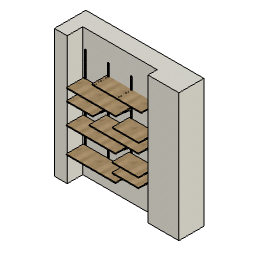
shelving_system (Autodesk Fusion 360 design; units mm, degrees)
Autodesk Fusion 360 part; units mm, degrees
note: some values were not read from the file. Chosen so that the rebuilt part matches the saved one: which face or edge a step refers to; the sign of a taper; where a step ends.
sketch "Sketch1" plane through (0, 0, 0) normal (0, 1, 0) x (1, 0, 0)
  line L0 (0, 0) -> (26, 0)
  line L1 (26, 0) -> (26, -1995)
  line L2 (26, -1995) -> (0, -1995)
  line L3 (0, -1995) -> (0, 0)
  dimension "d1" = 26
  dimension "d2" = 1995
  constraint horizontal L0
  constraint vertical L1
  constraint horizontal L2
  constraint vertical L3
  constraint coincident L0.start L3.end
  measures "d1" distance of L0.start L0.end
  measures "d2" distance of L0.start L2.end
extrude "Extrude1" add sketch "Sketch1" along normal blind 12 makes body 1
sketch "Sketch2" plane through (0, 0, 0) normal (0, -1, 0) x (1, 0, 0)
  line L0 (26, 1995) -> (0, 1995)
  line L1 (0, 1995) -> (0, 0)
  line L2 (0, 0) -> (26, 0)
  line L3 (26, 0) -> (26, 1995)
  line L4 (6.3705, 1487.1399) -> (6.3705, 1462.1399)
  arc A0 (6.3705, 1462.1399) -> (9.3705, 1462.1399) centre (7.8705, 1462.1399) ccw
  line L5 (9.3705, 1462.1399) -> (9.3705, 1487.1399)
  arc A1 (9.3705, 1487.1399) -> (6.3705, 1487.1399) centre (7.8705, 1487.1399) ccw
  line L6 (7.8705, 1487.1399) -> (7.8705, 1462.1399) construction
  dimension "d5" = 3
  constraint tangent L4 A0
  constraint tangent A0 L5
  constraint parallel L4 L5
  constraint tangent L5 A1
  constraint tangent L4 A1
  constraint vertical L6
  measures "d5" diameter of A0
extrude "Extrude2" cut sketch "Sketch2" along normal up to far side of body 1 contours L4 A0 L5 A1 bodies 1
ref_plane "WorkPlane1" through (13, 6, 997.5) normal (-1, 0, 0) x (0, 0, 1)
mirror "Mirror1" about plane through (13, 6, 997.5) normal (-1, 0, 0) of "Extrude2"
pattern_linear "R-Pattern1" count 30 spacing 50 along (0, 0, -1) of 8 faces at (6.3705, 4, 1478.8066) (9.3705, 4, 1470.4732) (6.878, 8, 1461.0152) (6.878, 4, 1488.2646) (19.6295, 4, 1478.8066) (16.6295, 4, 1470.4732) (17.137, 8, 1488.2646) (19.122, 8, 1461.0152) on bodies 1
pattern_linear "R-Pattern3" count 11 spacing 50 along (0, 0, 1) of 8 faces at (6.878, 4, 1488.2646) (6.3705, 4, 1478.8066) (9.3705, 4, 1470.4732) (17.137, 8, 1488.2646) (6.878, 8, 1461.0152) (19.6295, 4, 1478.8066) (16.6295, 4, 1470.4732) (19.122, 8, 1461.0152) on bodies 1
pattern_linear "R-Pattern2" count 4 spacing 500 along (1, 0, 0) of bodies 1 makes body 2 at (511.5402, 0, 3.6136) makes body 3 at (1011.5402, 0, 3.6136) makes body 4 at (1511.5402, 0, 3.6136)
sketch "Sketch3" plane through (0, 0, 0) normal (0, -1, 0) x (1, 0, 0)
  line L0 (16.6295, 12.1399) -> (16.6295, 37.1399)
  arc A0 (19.6295, 37.1399) -> (16.6295, 37.1399) centre (18.1295, 37.1399) ccw
  line L1 (19.6295, 37.1399) -> (19.6295, 12.1399)
  arc A1 (16.6295, 12.1399) -> (19.6295, 12.1399) centre (18.1295, 12.1399) ccw
  line L2 (16.6295, 62.1399) -> (16.6295, 87.1399)
  arc A2 (19.6295, 87.1399) -> (16.6295, 87.1399) centre (18.1295, 87.1399) ccw
  line L3 (19.6295, 87.1399) -> (19.6295, 62.1399)
  arc A3 (16.6295, 62.1399) -> (19.6295, 62.1399) centre (18.1295, 62.1399) ccw
  line L4 (16.6295, 112.1399) -> (16.6295, 137.1399)
  arc A4 (19.6295, 137.1399) -> (16.6295, 137.1399) centre (18.1295, 137.1399) ccw
  line L5 (19.6295, 137.1399) -> (19.6295, 112.1399)
  arc A5 (16.6295, 112.1399) -> (19.6295, 112.1399) centre (18.1295, 112.1399) ccw
  line L6 (16.6295, 162.1399) -> (16.6295, 187.1399)
  arc A6 (19.6295, 187.1399) -> (16.6295, 187.1399) centre (18.1295, 187.1399) ccw
  line L7 (19.6295, 187.1399) -> (19.6295, 162.1399)
  arc A7 (16.6295, 162.1399) -> (19.6295, 162.1399) centre (18.1295, 162.1399) ccw
  line L8 (16.6295, 212.1399) -> (16.6295, 237.1399)
  arc A8 (19.6295, 237.1399) -> (16.6295, 237.1399) centre (18.1295, 237.1399) ccw
  line L9 (19.6295, 237.1399) -> (19.6295, 212.1399)
  arc A9 (16.6295, 212.1399) -> (19.6295, 212.1399) centre (18.1295, 212.1399) ccw
  line L10 (16.6295, 262.1399) -> (16.6295, 287.1399)
  arc A10 (19.6295, 287.1399) -> (16.6295, 287.1399) centre (18.1295, 287.1399) ccw
  line L11 (19.6295, 287.1399) -> (19.6295, 262.1399)
  arc A11 (16.6295, 262.1399) -> (19.6295, 262.1399) centre (18.1295, 262.1399) ccw
  line L12 (16.6295, 312.1399) -> (16.6295, 337.1399)
  arc A12 (19.6295, 337.1399) -> (16.6295, 337.1399) centre (18.1295, 337.1399) ccw
  line L13 (19.6295, 337.1399) -> (19.6295, 312.1399)
  arc A13 (16.6295, 312.1399) -> (19.6295, 312.1399) centre (18.1295, 312.1399) ccw
  line L14 (16.6295, 362.1399) -> (16.6295, 387.1399)
  arc A14 (19.6295, 387.1399) -> (16.6295, 387.1399) centre (18.1295, 387.1399) ccw
  line L15 (19.6295, 387.1399) -> (19.6295, 362.1399)
  arc A15 (16.6295, 362.1399) -> (19.6295, 362.1399) centre (18.1295, 362.1399) ccw
  line L16 (16.6295, 412.1399) -> (16.6295, 437.1399)
  arc A16 (19.6295, 437.1399) -> (16.6295, 437.1399) centre (18.1295, 437.1399) ccw
  line L17 (19.6295, 437.1399) -> (19.6295, 412.1399)
  arc A17 (16.6295, 412.1399) -> (19.6295, 412.1399) centre (18.1295, 412.1399) ccw
  line L18 (16.6295, 462.1399) -> (16.6295, 487.1399)
  arc A18 (19.6295, 487.1399) -> (16.6295, 487.1399) centre (18.1295, 487.1399) ccw
  line L19 (19.6295, 487.1399) -> (19.6295, 462.1399)
  arc A19 (16.6295, 462.1399) -> (19.6295, 462.1399) centre (18.1295, 462.1399) ccw
  line L20 (16.6295, 512.1399) -> (16.6295, 537.1399)
  arc A20 (19.6295, 537.1399) -> (16.6295, 537.1399) centre (18.1295, 537.1399) ccw
  line L21 (19.6295, 537.1399) -> (19.6295, 512.1399)
  arc A21 (16.6295, 512.1399) -> (19.6295, 512.1399) centre (18.1295, 512.1399) ccw
  line L22 (16.6295, 562.1399) -> (16.6295, 587.1399)
  arc A22 (19.6295, 587.1399) -> (16.6295, 587.1399) centre (18.1295, 587.1399) ccw
  line L23 (19.6295, 587.1399) -> (19.6295, 562.1399)
  arc A23 (16.6295, 562.1399) -> (19.6295, 562.1399) centre (18.1295, 562.1399) ccw
  line L24 (16.6295, 612.1399) -> (16.6295, 637.1399)
  arc A24 (19.6295, 637.1399) -> (16.6295, 637.1399) centre (18.1295, 637.1399) ccw
  line L25 (19.6295, 637.1399) -> (19.6295, 612.1399)
  arc A25 (16.6295, 612.1399) -> (19.6295, 612.1399) centre (18.1295, 612.1399) ccw
  line L26 (16.6295, 662.1399) -> (16.6295, 687.1399)
  arc A26 (19.6295, 687.1399) -> (16.6295, 687.1399) centre (18.1295, 687.1399) ccw
  line L27 (19.6295, 687.1399) -> (19.6295, 662.1399)
  arc A27 (16.6295, 662.1399) -> (19.6295, 662.1399) centre (18.1295, 662.1399) ccw
  line L28 (16.6295, 712.1399) -> (16.6295, 737.1399)
  arc A28 (19.6295, 737.1399) -> (16.6295, 737.1399) centre (18.1295, 737.1399) ccw
  line L29 (19.6295, 737.1399) -> (19.6295, 712.1399)
  arc A29 (16.6295, 712.1399) -> (19.6295, 712.1399) centre (18.1295, 712.1399) ccw
  line L30 (16.6295, 762.1399) -> (16.6295, 787.1399)
  arc A30 (19.6295, 787.1399) -> (16.6295, 787.1399) centre (18.1295, 787.1399) ccw
  line L31 (19.6295, 787.1399) -> (19.6295, 762.1399)
  arc A31 (16.6295, 762.1399) -> (19.6295, 762.1399) centre (18.1295, 762.1399) ccw
  line L32 (16.6295, 812.1399) -> (16.6295, 837.1399)
  arc A32 (19.6295, 837.1399) -> (16.6295, 837.1399) centre (18.1295, 837.1399) ccw
  line L33 (19.6295, 837.1399) -> (19.6295, 812.1399)
  arc A33 (16.6295, 812.1399) -> (19.6295, 812.1399) centre (18.1295, 812.1399) ccw
  line L34 (16.6295, 862.1399) -> (16.6295, 887.1399)
  arc A34 (19.6295, 887.1399) -> (16.6295, 887.1399) centre (18.1295, 887.1399) ccw
  line L35 (19.6295, 887.1399) -> (19.6295, 862.1399)
  arc A35 (16.6295, 862.1399) -> (19.6295, 862.1399) centre (18.1295, 862.1399) ccw
  line L36 (16.6295, 912.1399) -> (16.6295, 937.1399)
  arc A36 (19.6295, 937.1399) -> (16.6295, 937.1399) centre (18.1295, 937.1399) ccw
  line L37 (19.6295, 937.1399) -> (19.6295, 912.1399)
  arc A37 (16.6295, 912.1399) -> (19.6295, 912.1399) centre (18.1295, 912.1399) ccw
  line L38 (16.6295, 962.1399) -> (16.6295, 987.1399)
  arc A38 (19.6295, 987.1399) -> (16.6295, 987.1399) centre (18.1295, 987.1399) ccw
  line L39 (19.6295, 987.1399) -> (19.6295, 962.1399)
  arc A39 (16.6295, 962.1399) -> (19.6295, 962.1399) centre (18.1295, 962.1399) ccw
  line L40 (16.6295, 1012.1399) -> (16.6295, 1037.1399)
  arc A40 (19.6295, 1037.1399) -> (16.6295, 1037.1399) centre (18.1295, 1037.1399) ccw
  line L41 (19.6295, 1037.1399) -> (19.6295, 1012.1399)
  arc A41 (16.6295, 1012.1399) -> (19.6295, 1012.1399) centre (18.1295, 1012.1399) ccw
  line L42 (16.6295, 1062.1399) -> (16.6295, 1087.1399)
  arc A42 (19.6295, 1087.1399) -> (16.6295, 1087.1399) centre (18.1295, 1087.1399) ccw
  line L43 (19.6295, 1087.1399) -> (19.6295, 1062.1399)
  arc A43 (16.6295, 1062.1399) -> (19.6295, 1062.1399) centre (18.1295, 1062.1399) ccw
  line L44 (16.6295, 1112.1399) -> (16.6295, 1137.1399)
  arc A44 (19.6295, 1137.1399) -> (16.6295, 1137.1399) centre (18.1295, 1137.1399) ccw
  line L45 (19.6295, 1137.1399) -> (19.6295, 1112.1399)
  arc A45 (16.6295, 1112.1399) -> (19.6295, 1112.1399) centre (18.1295, 1112.1399) ccw
  line L46 (16.6295, 1162.1399) -> (16.6295, 1187.1399)
  arc A46 (19.6295, 1187.1399) -> (16.6295, 1187.1399) centre (18.1295, 1187.1399) ccw
  line L47 (19.6295, 1187.1399) -> (19.6295, 1162.1399)
  arc A47 (16.6295, 1162.1399) -> (19.6295, 1162.1399) centre (18.1295, 1162.1399) ccw
  line L48 (16.6295, 1212.1399) -> (16.6295, 1237.1399)
  arc A48 (19.6295, 1237.1399) -> (16.6295, 1237.1399) centre (18.1295, 1237.1399) ccw
  line L49 (19.6295, 1237.1399) -> (19.6295, 1212.1399)
  arc A49 (16.6295, 1212.1399) -> (19.6295, 1212.1399) centre (18.1295, 1212.1399) ccw
  line L50 (16.6295, 1262.1399) -> (16.6295, 1287.1399)
  arc A50 (19.6295, 1287.1399) -> (16.6295, 1287.1399) centre (18.1295, 1287.1399) ccw
  line L51 (19.6295, 1287.1399) -> (19.6295, 1262.1399)
  arc A51 (16.6295, 1262.1399) -> (19.6295, 1262.1399) centre (18.1295, 1262.1399) ccw
  line L52 (16.6295, 1312.1399) -> (16.6295, 1337.1399)
  arc A52 (19.6295, 1337.1399) -> (16.6295, 1337.1399) centre (18.1295, 1337.1399) ccw
  line L53 (19.6295, 1337.1399) -> (19.6295, 1312.1399)
  arc A53 (16.6295, 1312.1399) -> (19.6295, 1312.1399) centre (18.1295, 1312.1399) ccw
  line L54 (16.6295, 1362.1399) -> (16.6295, 1387.1399)
  arc A54 (19.6295, 1387.1399) -> (16.6295, 1387.1399) centre (18.1295, 1387.1399) ccw
  line L55 (19.6295, 1387.1399) -> (19.6295, 1362.1399)
  arc A55 (16.6295, 1362.1399) -> (19.6295, 1362.1399) centre (18.1295, 1362.1399) ccw
  line L56 (16.6295, 1412.1399) -> (16.6295, 1437.1399)
  arc A56 (19.6295, 1437.1399) -> (16.6295, 1437.1399) centre (18.1295, 1437.1399) ccw
  line L57 (19.6295, 1437.1399) -> (19.6295, 1412.1399)
  arc A57 (16.6295, 1412.1399) -> (19.6295, 1412.1399) centre (18.1295, 1412.1399) ccw
  line L58 (9.3705, 37.1399) -> (9.3705, 12.1399)
  arc A58 (6.3705, 12.1399) -> (9.3705, 12.1399) centre (7.8705, 12.1399) ccw
  line L59 (6.3705, 12.1399) -> (6.3705, 37.1399)
  arc A59 (9.3705, 37.1399) -> (6.3705, 37.1399) centre (7.8705, 37.1399) ccw
  line L60 (9.3705, 87.1399) -> (9.3705, 62.1399)
  arc A60 (6.3705, 62.1399) -> (9.3705, 62.1399) centre (7.8705, 62.1399) ccw
  line L61 (6.3705, 62.1399) -> (6.3705, 87.1399)
  arc A61 (9.3705, 87.1399) -> (6.3705, 87.1399) centre (7.8705, 87.1399) ccw
  line L62 (9.3705, 137.1399) -> (9.3705, 112.1399)
  arc A62 (6.3705, 112.1399) -> (9.3705, 112.1399) centre (7.8705, 112.1399) ccw
  line L63 (6.3705, 112.1399) -> (6.3705, 137.1399)
  arc A63 (9.3705, 137.1399) -> (6.3705, 137.1399) centre (7.8705, 137.1399) ccw
  line L64 (9.3705, 187.1399) -> (9.3705, 162.1399)
  arc A64 (6.3705, 162.1399) -> (9.3705, 162.1399) centre (7.8705, 162.1399) ccw
  line L65 (6.3705, 162.1399) -> (6.3705, 187.1399)
  arc A65 (9.3705, 187.1399) -> (6.3705, 187.1399) centre (7.8705, 187.1399) ccw
  line L66 (9.3705, 237.1399) -> (9.3705, 212.1399)
  arc A66 (6.3705, 212.1399) -> (9.3705, 212.1399) centre (7.8705, 212.1399) ccw
  line L67 (6.3705, 212.1399) -> (6.3705, 237.1399)
  arc A67 (9.3705, 237.1399) -> (6.3705, 237.1399) centre (7.8705, 237.1399) ccw
  line L68 (9.3705, 287.1399) -> (9.3705, 262.1399)
  arc A68 (6.3705, 262.1399) -> (9.3705, 262.1399) centre (7.8705, 262.1399) ccw
  line L69 (6.3705, 262.1399) -> (6.3705, 287.1399)
  arc A69 (9.3705, 287.1399) -> (6.3705, 287.1399) centre (7.8705, 287.1399) ccw
  line L70 (9.3705, 337.1399) -> (9.3705, 312.1399)
  arc A70 (6.3705, 312.1399) -> (9.3705, 312.1399) centre (7.8705, 312.1399) ccw
  line L71 (6.3705, 312.1399) -> (6.3705, 337.1399)
  arc A71 (9.3705, 337.1399) -> (6.3705, 337.1399) centre (7.8705, 337.1399) ccw
  line L72 (9.3705, 387.1399) -> (9.3705, 362.1399)
  arc A72 (6.3705, 362.1399) -> (9.3705, 362.1399) centre (7.8705, 362.1399) ccw
  line L73 (6.3705, 362.1399) -> (6.3705, 387.1399)
  arc A73 (9.3705, 387.1399) -> (6.3705, 387.1399) centre (7.8705, 387.1399) ccw
  line L74 (9.3705, 437.1399) -> (9.3705, 412.1399)
  arc A74 (6.3705, 412.1399) -> (9.3705, 412.1399) centre (7.8705, 412.1399) ccw
  line L75 (6.3705, 412.1399) -> (6.3705, 437.1399)
  arc A75 (9.3705, 437.1399) -> (6.3705, 437.1399) centre (7.8705, 437.1399) ccw
  line L76 (9.3705, 487.1399) -> (9.3705, 462.1399)
  arc A76 (6.3705, 462.1399) -> (9.3705, 462.1399) centre (7.8705, 462.1399) ccw
  line L77 (6.3705, 462.1399) -> (6.3705, 487.1399)
  arc A77 (9.3705, 487.1399) -> (6.3705, 487.1399) centre (7.8705, 487.1399) ccw
  line L78 (9.3705, 537.1399) -> (9.3705, 512.1399)
  arc A78 (6.3705, 512.1399) -> (9.3705, 512.1399) centre (7.8705, 512.1399) ccw
  line L79 (6.3705, 512.1399) -> (6.3705, 537.1399)
  arc A79 (9.3705, 537.1399) -> (6.3705, 537.1399) centre (7.8705, 537.1399) ccw
  line L80 (9.3705, 587.1399) -> (9.3705, 562.1399)
  arc A80 (6.3705, 562.1399) -> (9.3705, 562.1399) centre (7.8705, 562.1399) ccw
  line L81 (6.3705, 562.1399) -> (6.3705, 587.1399)
  arc A81 (9.3705, 587.1399) -> (6.3705, 587.1399) centre (7.8705, 587.1399) ccw
  line L82 (9.3705, 637.1399) -> (9.3705, 612.1399)
  arc A82 (6.3705, 612.1399) -> (9.3705, 612.1399) centre (7.8705, 612.1399) ccw
  line L83 (6.3705, 612.1399) -> (6.3705, 637.1399)
  arc A83 (9.3705, 637.1399) -> (6.3705, 637.1399) centre (7.8705, 637.1399) ccw
  line L84 (9.3705, 687.1399) -> (9.3705, 662.1399)
  arc A84 (6.3705, 662.1399) -> (9.3705, 662.1399) centre (7.8705, 662.1399) ccw
  line L85 (6.3705, 662.1399) -> (6.3705, 687.1399)
  arc A85 (9.3705, 687.1399) -> (6.3705, 687.1399) centre (7.8705, 687.1399) ccw
  line L86 (9.3705, 737.1399) -> (9.3705, 712.1399)
  arc A86 (6.3705, 712.1399) -> (9.3705, 712.1399) centre (7.8705, 712.1399) ccw
  line L87 (6.3705, 712.1399) -> (6.3705, 737.1399)
  arc A87 (9.3705, 737.1399) -> (6.3705, 737.1399) centre (7.8705, 737.1399) ccw
  line L88 (9.3705, 787.1399) -> (9.3705, 762.1399)
  arc A88 (6.3705, 762.1399) -> (9.3705, 762.1399) centre (7.8705, 762.1399) ccw
  line L89 (6.3705, 762.1399) -> (6.3705, 787.1399)
  arc A89 (9.3705, 787.1399) -> (6.3705, 787.1399) centre (7.8705, 787.1399) ccw
  line L90 (9.3705, 837.1399) -> (9.3705, 812.1399)
  arc A90 (6.3705, 812.1399) -> (9.3705, 812.1399) centre (7.8705, 812.1399) ccw
  line L91 (6.3705, 812.1399) -> (6.3705, 837.1399)
  arc A91 (9.3705, 837.1399) -> (6.3705, 837.1399) centre (7.8705, 837.1399) ccw
  line L92 (9.3705, 887.1399) -> (9.3705, 862.1399)
  arc A92 (6.3705, 862.1399) -> (9.3705, 862.1399) centre (7.8705, 862.1399) ccw
  line L93 (6.3705, 862.1399) -> (6.3705, 887.1399)
  arc A93 (9.3705, 887.1399) -> (6.3705, 887.1399) centre (7.8705, 887.1399) ccw
  line L94 (9.3705, 937.1399) -> (9.3705, 912.1399)
  arc A94 (6.3705, 912.1399) -> (9.3705, 912.1399) centre (7.8705, 912.1399) ccw
  line L95 (6.3705, 912.1399) -> (6.3705, 937.1399)
  arc A95 (9.3705, 937.1399) -> (6.3705, 937.1399) centre (7.8705, 937.1399) ccw
  line L96 (9.3705, 987.1399) -> (9.3705, 962.1399)
  arc A96 (6.3705, 962.1399) -> (9.3705, 962.1399) centre (7.8705, 962.1399) ccw
  line L97 (6.3705, 962.1399) -> (6.3705, 987.1399)
  arc A97 (9.3705, 987.1399) -> (6.3705, 987.1399) centre (7.8705, 987.1399) ccw
  line L98 (9.3705, 1037.1399) -> (9.3705, 1012.1399)
  arc A98 (6.3705, 1012.1399) -> (9.3705, 1012.1399) centre (7.8705, 1012.1399) ccw
  line L99 (6.3705, 1012.1399) -> (6.3705, 1037.1399)
  arc A99 (9.3705, 1037.1399) -> (6.3705, 1037.1399) centre (7.8705, 1037.1399) ccw
  line L100 (9.3705, 1087.1399) -> (9.3705, 1062.1399)
  arc A100 (6.3705, 1062.1399) -> (9.3705, 1062.1399) centre (7.8705, 1062.1399) ccw
  line L101 (6.3705, 1062.1399) -> (6.3705, 1087.1399)
  arc A101 (9.3705, 1087.1399) -> (6.3705, 1087.1399) centre (7.8705, 1087.1399) ccw
  line L102 (9.3705, 1137.1399) -> (9.3705, 1112.1399)
  arc A102 (6.3705, 1112.1399) -> (9.3705, 1112.1399) centre (7.8705, 1112.1399) ccw
  line L103 (6.3705, 1112.1399) -> (6.3705, 1137.1399)
  arc A103 (9.3705, 1137.1399) -> (6.3705, 1137.1399) centre (7.8705, 1137.1399) ccw
  line L104 (9.3705, 1187.1399) -> (9.3705, 1162.1399)
  arc A104 (6.3705, 1162.1399) -> (9.3705, 1162.1399) centre (7.8705, 1162.1399) ccw
  line L105 (6.3705, 1162.1399) -> (6.3705, 1187.1399)
  arc A105 (9.3705, 1187.1399) -> (6.3705, 1187.1399) centre (7.8705, 1187.1399) ccw
  line L106 (9.3705, 1237.1399) -> (9.3705, 1212.1399)
  arc A106 (6.3705, 1212.1399) -> (9.3705, 1212.1399) centre (7.8705, 1212.1399) ccw
  line L107 (6.3705, 1212.1399) -> (6.3705, 1237.1399)
  arc A107 (9.3705, 1237.1399) -> (6.3705, 1237.1399) centre (7.8705, 1237.1399) ccw
  line L108 (9.3705, 1287.1399) -> (9.3705, 1262.1399)
  arc A108 (6.3705, 1262.1399) -> (9.3705, 1262.1399) centre (7.8705, 1262.1399) ccw
  line L109 (6.3705, 1262.1399) -> (6.3705, 1287.1399)
  arc A109 (9.3705, 1287.1399) -> (6.3705, 1287.1399) centre (7.8705, 1287.1399) ccw
  line L110 (9.3705, 1337.1399) -> (9.3705, 1312.1399)
  arc A110 (6.3705, 1312.1399) -> (9.3705, 1312.1399) centre (7.8705, 1312.1399) ccw
  line L111 (6.3705, 1312.1399) -> (6.3705, 1337.1399)
  arc A111 (9.3705, 1337.1399) -> (6.3705, 1337.1399) centre (7.8705, 1337.1399) ccw
  line L112 (9.3705, 1387.1399) -> (9.3705, 1362.1399)
  arc A112 (6.3705, 1362.1399) -> (9.3705, 1362.1399) centre (7.8705, 1362.1399) ccw
  line L113 (6.3705, 1362.1399) -> (6.3705, 1387.1399)
  arc A113 (9.3705, 1387.1399) -> (6.3705, 1387.1399) centre (7.8705, 1387.1399) ccw
  line L114 (9.3705, 1437.1399) -> (9.3705, 1412.1399)
  arc A114 (6.3705, 1412.1399) -> (9.3705, 1412.1399) centre (7.8705, 1412.1399) ccw
  line L115 (6.3705, 1412.1399) -> (6.3705, 1437.1399)
  arc A115 (9.3705, 1437.1399) -> (6.3705, 1437.1399) centre (7.8705, 1437.1399) ccw
  line L116 (16.6295, 1462.1399) -> (16.6295, 1487.1399)
  arc A116 (19.6295, 1487.1399) -> (16.6295, 1487.1399) centre (18.1295, 1487.1399) ccw
  line L117 (19.6295, 1487.1399) -> (19.6295, 1462.1399)
  arc A117 (16.6295, 1462.1399) -> (19.6295, 1462.1399) centre (18.1295, 1462.1399) ccw
  line L118 (9.3705, 1487.1399) -> (9.3705, 1462.1399)
  arc A118 (6.3705, 1462.1399) -> (9.3705, 1462.1399) centre (7.8705, 1462.1399) ccw
  line L119 (6.3705, 1462.1399) -> (6.3705, 1487.1399)
  arc A119 (9.3705, 1487.1399) -> (6.3705, 1487.1399) centre (7.8705, 1487.1399) ccw
  line L120 (26, 1995) -> (0, 1995)
  line L121 (0, 1995) -> (0, 0)
  line L122 (0, 0) -> (26, 0)
  line L123 (26, 0) -> (26, 1995)
  line L124 (30, 80) -> (50, 80)
  line L125 (50, 80) -> (50, 10.1178)
  line L126 (50, 10.1178) -> (30, 10.1178)
  line L127 (30, 10.1178) -> (30, 80)
  line L128 (16.6295, 1962.1399) -> (16.6295, 1987.1399)
  arc A120 (19.6295, 1987.1399) -> (16.6295, 1987.1399) centre (18.1295, 1987.1399) ccw
  line L129 (19.6295, 1987.1399) -> (19.6295, 1962.1399)
  arc A121 (16.6295, 1962.1399) -> (19.6295, 1962.1399) centre (18.1295, 1962.1399) ccw
  line L130 (16.6295, 1912.1399) -> (16.6295, 1937.1399)
  arc A122 (19.6295, 1937.1399) -> (16.6295, 1937.1399) centre (18.1295, 1937.1399) ccw
  line L131 (19.6295, 1937.1399) -> (19.6295, 1912.1399)
  arc A123 (16.6295, 1912.1399) -> (19.6295, 1912.1399) centre (18.1295, 1912.1399) ccw
  line L132 (16.6295, 1862.1399) -> (16.6295, 1887.1399)
  arc A124 (19.6295, 1887.1399) -> (16.6295, 1887.1399) centre (18.1295, 1887.1399) ccw
  line L133 (19.6295, 1887.1399) -> (19.6295, 1862.1399)
  arc A125 (16.6295, 1862.1399) -> (19.6295, 1862.1399) centre (18.1295, 1862.1399) ccw
  line L134 (16.6295, 1812.1399) -> (16.6295, 1837.1399)
  arc A126 (19.6295, 1837.1399) -> (16.6295, 1837.1399) centre (18.1295, 1837.1399) ccw
  line L135 (19.6295, 1837.1399) -> (19.6295, 1812.1399)
  arc A127 (16.6295, 1812.1399) -> (19.6295, 1812.1399) centre (18.1295, 1812.1399) ccw
  line L136 (16.6295, 1762.1399) -> (16.6295, 1787.1399)
  arc A128 (19.6295, 1787.1399) -> (16.6295, 1787.1399) centre (18.1295, 1787.1399) ccw
  line L137 (19.6295, 1787.1399) -> (19.6295, 1762.1399)
  arc A129 (16.6295, 1762.1399) -> (19.6295, 1762.1399) centre (18.1295, 1762.1399) ccw
  line L138 (16.6295, 1712.1399) -> (16.6295, 1737.1399)
  arc A130 (19.6295, 1737.1399) -> (16.6295, 1737.1399) centre (18.1295, 1737.1399) ccw
  line L139 (19.6295, 1737.1399) -> (19.6295, 1712.1399)
  arc A131 (16.6295, 1712.1399) -> (19.6295, 1712.1399) centre (18.1295, 1712.1399) ccw
  line L140 (16.6295, 1662.1399) -> (16.6295, 1687.1399)
  arc A132 (19.6295, 1687.1399) -> (16.6295, 1687.1399) centre (18.1295, 1687.1399) ccw
  line L141 (19.6295, 1687.1399) -> (19.6295, 1662.1399)
  arc A133 (16.6295, 1662.1399) -> (19.6295, 1662.1399) centre (18.1295, 1662.1399) ccw
  line L142 (16.6295, 1612.1399) -> (16.6295, 1637.1399)
  arc A134 (19.6295, 1637.1399) -> (16.6295, 1637.1399) centre (18.1295, 1637.1399) ccw
  line L143 (19.6295, 1637.1399) -> (19.6295, 1612.1399)
  arc A135 (16.6295, 1612.1399) -> (19.6295, 1612.1399) centre (18.1295, 1612.1399) ccw
  line L144 (16.6295, 1562.1399) -> (16.6295, 1587.1399)
  arc A136 (19.6295, 1587.1399) -> (16.6295, 1587.1399) centre (18.1295, 1587.1399) ccw
  line L145 (19.6295, 1587.1399) -> (19.6295, 1562.1399)
  arc A137 (16.6295, 1562.1399) -> (19.6295, 1562.1399) centre (18.1295, 1562.1399) ccw
  line L146 (16.6295, 1512.1399) -> (16.6295, 1537.1399)
  arc A138 (19.6295, 1537.1399) -> (16.6295, 1537.1399) centre (18.1295, 1537.1399) ccw
  line L147 (19.6295, 1537.1399) -> (19.6295, 1512.1399)
  arc A139 (16.6295, 1512.1399) -> (19.6295, 1512.1399) centre (18.1295, 1512.1399) ccw
  line L148 (9.3705, 1987.1399) -> (9.3705, 1962.1399)
  arc A140 (6.3705, 1962.1399) -> (9.3705, 1962.1399) centre (7.8705, 1962.1399) ccw
  line L149 (6.3705, 1962.1399) -> (6.3705, 1987.1399)
  arc A141 (9.3705, 1987.1399) -> (6.3705, 1987.1399) centre (7.8705, 1987.1399) ccw
  line L150 (9.3705, 1937.1399) -> (9.3705, 1912.1399)
  arc A142 (6.3705, 1912.1399) -> (9.3705, 1912.1399) centre (7.8705, 1912.1399) ccw
  line L151 (6.3705, 1912.1399) -> (6.3705, 1937.1399)
  arc A143 (9.3705, 1937.1399) -> (6.3705, 1937.1399) centre (7.8705, 1937.1399) ccw
  line L152 (9.3705, 1887.1399) -> (9.3705, 1862.1399)
  arc A144 (6.3705, 1862.1399) -> (9.3705, 1862.1399) centre (7.8705, 1862.1399) ccw
  line L153 (6.3705, 1862.1399) -> (6.3705, 1887.1399)
  arc A145 (9.3705, 1887.1399) -> (6.3705, 1887.1399) centre (7.8705, 1887.1399) ccw
  line L154 (9.3705, 1837.1399) -> (9.3705, 1812.1399)
  arc A146 (6.3705, 1812.1399) -> (9.3705, 1812.1399) centre (7.8705, 1812.1399) ccw
  line L155 (6.3705, 1812.1399) -> (6.3705, 1837.1399)
  arc A147 (9.3705, 1837.1399) -> (6.3705, 1837.1399) centre (7.8705, 1837.1399) ccw
  line L156 (9.3705, 1787.1399) -> (9.3705, 1762.1399)
  arc A148 (6.3705, 1762.1399) -> (9.3705, 1762.1399) centre (7.8705, 1762.1399) ccw
  line L157 (6.3705, 1762.1399) -> (6.3705, 1787.1399)
  arc A149 (9.3705, 1787.1399) -> (6.3705, 1787.1399) centre (7.8705, 1787.1399) ccw
  line L158 (9.3705, 1737.1399) -> (9.3705, 1712.1399)
  arc A150 (6.3705, 1712.1399) -> (9.3705, 1712.1399) centre (7.8705, 1712.1399) ccw
  line L159 (6.3705, 1712.1399) -> (6.3705, 1737.1399)
  arc A151 (9.3705, 1737.1399) -> (6.3705, 1737.1399) centre (7.8705, 1737.1399) ccw
  line L160 (9.3705, 1687.1399) -> (9.3705, 1662.1399)
  arc A152 (6.3705, 1662.1399) -> (9.3705, 1662.1399) centre (7.8705, 1662.1399) ccw
  line L161 (6.3705, 1662.1399) -> (6.3705, 1687.1399)
  arc A153 (9.3705, 1687.1399) -> (6.3705, 1687.1399) centre (7.8705, 1687.1399) ccw
  line L162 (9.3705, 1637.1399) -> (9.3705, 1612.1399)
  arc A154 (6.3705, 1612.1399) -> (9.3705, 1612.1399) centre (7.8705, 1612.1399) ccw
  line L163 (6.3705, 1612.1399) -> (6.3705, 1637.1399)
  arc A155 (9.3705, 1637.1399) -> (6.3705, 1637.1399) centre (7.8705, 1637.1399) ccw
  line L164 (9.3705, 1587.1399) -> (9.3705, 1562.1399)
  arc A156 (6.3705, 1562.1399) -> (9.3705, 1562.1399) centre (7.8705, 1562.1399) ccw
  line L165 (6.3705, 1562.1399) -> (6.3705, 1587.1399)
  arc A157 (9.3705, 1587.1399) -> (6.3705, 1587.1399) centre (7.8705, 1587.1399) ccw
  line L166 (9.3705, 1537.1399) -> (9.3705, 1512.1399)
  arc A158 (6.3705, 1512.1399) -> (9.3705, 1512.1399) centre (7.8705, 1512.1399) ccw
  line L167 (6.3705, 1512.1399) -> (6.3705, 1537.1399)
  arc A159 (9.3705, 1537.1399) -> (6.3705, 1537.1399) centre (7.8705, 1537.1399) ccw
  constraint horizontal L124
  constraint vertical L125
  constraint horizontal L126
  constraint vertical L127
extrude "Extrude3" add sketch "Sketch3" along normal blind 370 separate body contours L124 L125 L126 L127 makes body 5
draft "Draft1" angle 10 neutral plane through (0, 0, 0) pull (0, -1, 0) 1 faces at (43.3333, -123.3333, 10.1178) on bodies 5
move_body "Align1" bodies 5 to x (1, 0, 0) y (0, 1, 0) z (0, 0, 1) at (-27, 0, 0)
move_body "Move1" bodies 5 to x (1, 0, 0) y (0, 1, 0) z (0, 0, 1) at (0, 0, 150)
copy_body "CopyPasteBodies1" bodies 5 makes body 6
move_body "Move2" bodies 6 to x (1, 0, 0) y (0, 1, 0) z (0, 0, 1) at (0, 0, 600)
copy_body "CopyPasteBodies2" bodies 6 makes body 7
move_body "Move3" bodies 7 to x (1, 0, 0) y (0, 1, 0) z (0, 0, 1) at (0, 0, 400)
copy_body "CopyPasteBodies3" bodies 7 makes body 8
move_body "Move4" bodies 8 to x (1, 0, 0) y (0, 1, 0) z (0, 0, 1) at (0, 0, 200)
move_body "Move5" bodies 6 to x (1, 0, 0) y (0, 1, 0) z (0, 0, 1) at (0, 0, -50)
move_body "Move6" bodies 7 to x (1, 0, 0) y (0, 1, 0) z (0, 0, 1) at (0, 0, -50)
copy_body "CopyPasteBodies4" bodies 5 makes body 9
move_body "Move7" bodies 9 to x (1, 0, 0) y (0, 1, 0) z (0, 0, 1) at (500, 0, 0)
copy_body "CopyPasteBodies5" bodies 9 makes body 10
move_body "Move8" bodies 10 to x (1, 0, 0) y (0, 1, 0) z (0, 0, 1) at (500, 0, 0)
copy_body "CopyPasteBodies6" bodies 6 makes body 11
move_body "Move9" bodies 11 to x (1, 0, 0) y (0, 1, 0) z (0, 0, 1) at (500, 0, 0)
copy_body "CopyPasteBodies7" bodies 11 makes body 12
move_body "Move10" bodies 12 to x (1, 0, 0) y (0, 1, 0) z (0, 0, 1) at (500, 0, 0)
copy_body "CopyPasteBodies8" bodies 7 makes body 13
move_body "Move11" bodies 13 to x (1, 0, 0) y (0, 1, 0) z (0, 0, 1) at (500, 0, 0)
copy_body "CopyPasteBodies9" bodies 8 makes body 14
move_body "Move12" bodies 14 to x (1, 0, 0) y (0, 1, 0) z (0, 0, 1) at (500, 0, 0)
copy_body "CopyPasteBodies10" bodies 12 makes body 15
move_body "Move13" bodies 15 to x (1, 0, 0) y (0, 1, 0) z (0, 0, 1) at (0, 0, 250)
copy_body "CopyPasteBodies11" bodies 15 makes body 16
move_body "Move14" bodies 16 to x (1, 0, 0) y (0, 1, 0) z (0, 0, 1) at (500, 0, 0)
copy_body "CopyPasteBodies12" bodies 15 makes body 17
move_body "Move15" bodies 17 to x (1, 0, 0) y (0, 1, 0) z (0, 0, 1) at (-500, 0, 0)
move_body "Move16" bodies 5 9 10 to x (1, 0, 0) y (0, 1, 0) z (0, 0, 1) at (0, -8.6824, -49.2404)
move_body "Move17" bodies 6 11 15 17 12 16 to x (1, 0, 0) y (0, 1, 0) z (0, 0, 1) at (0, -8.6824, -49.2404)
copy_body "CopyPasteBodies13" bodies 14 makes body 18
move_body "Move18" bodies 18 to x (1, 0, 0) y (0, 1, 0) z (0, 0, 1) at (500, 0, 0)
copy_body "CopyPasteBodies14" bodies 13 makes body 19
move_body "Move19" bodies 19 to x (1, 0, 0) y (0, 1, 0) z (0, 0, 1) at (500, 0, 0)
copy_body "CopyPasteBodies15" bodies 19 makes body 20
move_body "Move20" bodies 20 to x (1, 0, 0) y (0, 1, 0) z (0, 0, 1) at (500, 0, 0)
copy_body "CopyPasteBodies16" bodies 12 makes body 21
move_body "Move21" bodies 21 to x (1, 0, 0) y (0, 1, 0) z (0, 0, 1) at (0, 0, -200)
copy_body "CopyPasteBodies17" bodies 21 makes body 22
move_body "Move22" bodies 22 to x (1, 0, 0) y (0, 1, 0) z (0, 0, 1) at (0, 0, -200)
copy_body "CopyPasteBodies18" bodies 21 makes body 23
move_body "Move23" bodies 23 to x (1, 0, 0) y (0, 1, 0) z (0, 0, 1) at (500, 0, 0)
copy_body "CopyPasteBodies19" bodies 22 makes body 24
move_body "Move24" bodies 24 to x (1, 0, 0) y (0, 1, 0) z (0, 0, 1) at (500, 0, 0)
sketch "Sketch4" plane through (0, 0, 0) normal (0, 0, 1) x (1, 0, 0)
  line L0 (-25, -375) -> (550, -375)
  line L1 (550, -375) -> (550, -1.9041)
  line L2 (550, -1.9041) -> (-25, -1.9041)
  line L3 (-25, -1.9041) -> (-25, -375)
  constraint horizontal L0
  constraint vertical L1
  constraint horizontal L2
  constraint vertical L3
extrude "Extrude4" add sketch "Sketch4" along normal blind 20 separate body makes body 25
move_body "Move25" bodies 25 to x (1, 0, 0) y (0, 1, 0) z (0, 0, 1) at (0, 0, 1200)
move_body "Move26" bodies 25 to x (1, 0, 0) y (0, 1, 0) z (0, 0, 1) at (28, 3.452, -20)
move_body "Move27" bodies 25 to x (1, 0, 0) y (0, 1, 0) z (0, 0, 1) at (-25, 0, 0)
sketch "Sketch5" plane through (0, 0, 0) normal (0, 0, 1) x (1, 0, 0)
  line L0 (1550, -2.2279) -> (475, -2.2279)
  line L1 (475, -2.2279) -> (475, -375)
  line L2 (475, -375) -> (1550, -375)
  line L3 (1550, -375) -> (1550, -2.2279)
  constraint horizontal L0
  constraint vertical L1
  constraint horizontal L2
  constraint vertical L3
extrude "Extrude5" add sketch "Sketch5" along normal blind 20 separate body makes body 26
move_body "Move28" bodies 26 to x (1, 0, 0) y (0, 1, 0) z (0, 0, 1) at (28, -3.6824, 980.7596)
move_body "Move29" bodies 26 to x (1, 0, 0) y (0, 1, 0) z (0, 0, 1) at (-25, 0, 0)
copy_body "CopyPasteBodies20" bodies 26 makes body 27
move_body "Move30" bodies 27 to x (1, 0, 0) y (0, 1, 0) z (0, 0, 1) at (-475, 8.6824, 449.2404)
move_body "Move31" bodies 27 to x (1, 0, 0) y (0, 1, 0) z (0, 0, 1) at (-25, 0, 0)
copy_body "CopyPasteBodies21" bodies 25 makes body 28
move_body "Move32" bodies 28 to x (1, 0, 0) y (0, 1, 0) z (0, 0, 1) at (1000, 0, 0)
copy_body "CopyPasteBodies22" bodies 27 makes body 29
move_body "Move33" bodies 29 to x (1, 0, 0) y (0, 1, 0) z (0, 0, 1) at (25, -8.6824, -699.2404)
move_body "Move34" bodies 29 to x (1, 0, 0) y (0, 1, 0) z (0, 0, 1) at (-25, 0, 0)
copy_body "CopyPasteBodies23" bodies 29 makes body 30
move_body "Move35" bodies 30 to x (1, 0, 0) y (0, 1, 0) z (0, 0, 1) at (25, 0, -550)
move_body "Move36" bodies 30 to x (1, 0, 0) y (0, 1, 0) z (0, 0, 1) at (-25, 0, 0)
copy_body "CopyPasteBodies24" bodies 28 makes body 31
move_body "Move37" bodies 31 to x (1, 0, 0) y (0, 1, 0) z (0, 0, 1) at (25, -7.1345, -649.2404)
move_body "Move38" bodies 31 to x (1, 0, 0) y (0, 1, 0) z (0, 0, 1) at (-25, 0, 0)
copy_body "CopyPasteBodies25" bodies 31 makes body 32
move_body "Move39" bodies 32 to x (1, 0, 0) y (0, 1, 0) z (0, 0, 1) at (25, 0, -200)
move_body "Move40" bodies 32 to x (1, 0, 0) y (0, 1, 0) z (0, 0, 1) at (-25, 0, 0)
sketch "Sketch6" plane through (0, 0, 0) normal (0, 0, 1) x (1, 0, 0)
  line L0 (0, 609.9461) -> (1620, 609.9461)
  line L1 (1620, 609.9461) -> (1620, 955.2191)
  line L2 (1620, 955.2191) -> (0, 955.2191)
  line L3 (0, 955.2191) -> (0, 609.9461)
  line L4 (0, 955.2191) -> (-277.9423, 955.2191)
  line L5 (-277.9423, 955.2191) -> (-277.9423, 270.2191)
  line L6 (-277.9423, 270.2191) -> (0, 270.2191)
  line L7 (0, 270.2191) -> (0, 955.2191)
  line L8 (1620, 955.2191) -> (2292.1723, 955.2191)
  line L9 (2292.1723, 955.2191) -> (2292.1723, 410.2191)
  line L10 (2292.1723, 410.2191) -> (1620, 410.2191)
  line L11 (1620, 410.2191) -> (1620, 955.2191)
  dimension "d26" = 1620
  dimension "d27" = 685
  dimension "d28" = 545
  constraint horizontal L0
  constraint vertical L1
  constraint horizontal L2
  constraint vertical L3
  constraint horizontal L4
  constraint vertical L5
  constraint horizontal L6
  constraint vertical L7
  constraint horizontal L8
  constraint vertical L9
  constraint horizontal L10
  constraint vertical L11
  measures "d26" distance of L0.start L0.end
  measures "d27" distance of L2.end L6.end
  measures "d28" distance of L1.end L10.end
extrude "Extrude6" add sketch "Sketch6" along normal blind 2790 separate body makes body 33
move_body "Move41" bodies 20 5 31 16 9 32 26 14 25 7 21 1 19 8 17 15 13 29 23 11 4 24 3 6 12 18 2 10 22 28 30 27 to x (1, 0, 0) y (0, 1, 0) z (0, 0, 1) at (0, -1000, 0)
ref_plane "WorkPlane2" through (810, 510.0826, 1395) normal (-1, 0, 0) x (0, -1, 0)
move_body "Move42" bodies 6 10 12 17 25 26 9 14 21 20 24 32 13 11 28 18 19 29 16 22 15 23 8 30 2 7 3 1 31 4 5 27 to x (1, 0, 0) y (0, 1, 0) z (0, 0, 1) at (0, 1597.9461, 0)
move_body "Move43" bodies 28 13 9 22 29 18 16 32 19 17 24 21 20 14 1 4 31 25 26 5 3 27 7 11 6 10 12 30 15 23 2 8 to x (1, 0, 0) y (0, 1, 0) z (0, 0, 1) at (50, 0, 0)
move_body "Move44" bodies 28 13 9 22 29 18 16 32 19 17 24 21 20 14 1 4 31 25 26 5 3 27 7 11 6 10 12 30 15 23 2 8 to x (1, 0, 0) y (0, 1, 0) z (0, 0, 1) at (0, 0, 400)
copy_body "CopyPasteBodies26" bodies 18 makes body 34
move_body "Move45" bodies 34 to x (1, 0, 0) y (0, 1, 0) z (0, 0, 1) at (0, 52.0945, 295.4423)
copy_body "CopyPasteBodies27" bodies 14 makes body 35
move_body "Move46" bodies 35 to x (1, 0, 0) y (0, 1, 0) z (0, 0, 1) at (0, 52.0945, 295.4423)
copy_body "CopyPasteBodies28" bodies 20 makes body 36
move_body "Move47" bodies 36 to x (1, 0, 0) y (0, 1, 0) z (0, 0, 1) at (0, 95.5065, 541.6443)
copy_body "CopyPasteBodies29" bodies 27 makes body 37
move_body "Move48" bodies 37 to x (1, 0, 0) y (0, 1, 0) z (0, 0, 1) at (525, 52.0945, 290.8011)
move_body "Move49" bodies 37 to x (1, 0, 0) y (0, 1, 0) z (0, 0, 1) at (-25, 0, 0)
